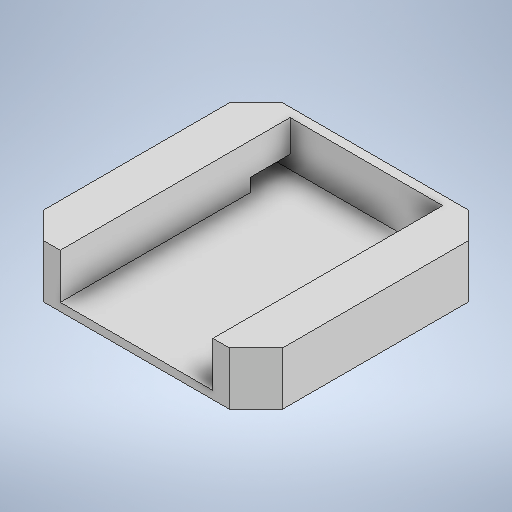
# Autodesk Inventor part: console case
Saved by Autodesk Inventor 2025.3 (Build 293356030, 356C)
## iProperties
Created: 2026-02-07
Part Number: console case
Material: Generic
Document SubType Name: Modeling
Designer: Adams
Density: 1 g/cm^3
Appearance: Default
Author: Adams
Autodesk Inventor part; units mm, degrees
ref_plane "YZ Plane" through (0, 0, 0) normal (1, 0, 0) x (0, 1, 0)
ref_plane "XZ Plane" through (0, 0, 0) normal (0, 1, 0) x (-1, 0, 0)
ref_plane "XY Plane" through (0, 0, 0) normal (0, 0, 1) x (1, 0, 0)
sketch "Sketch1" plane through (0, 0, 0) normal (0, 1, 0) x (-1, 0, 0)
  line L0 (28.75, 45) -> (-28.75, 45) construction
  line L1 (-28.75, 45) -> (-28.75, -41.6)
  line L2 (-28.75, -41.6) -> (28.75, -41.6)
  line L3 (28.75, -41.6) -> (28.75, 45)
  line L4 (28.75, 45) -> (-28.75, -41.6) construction
  line L5 (-28.75, 45) -> (28.75, -41.6) construction
  line L6 (45, 45) -> (-45, 45)
  line L7 (-45, 45) -> (-45, -45)
  line L8 (-45, -45) -> (45, -45)
  line L9 (45, -45) -> (45, 45)
  line L10 (45, 45) -> (-45, -45) construction
  line L11 (-45, 45) -> (45, -45) construction
  point P0 (0, 0)
  point P1 (0, 1.7)
  point P2 (28.75, 45)
  dimension "d0" = 57.5
  dimension "d1" = 86.6
  dimension "d2" = 90
  dimension "d3" = 90
  dimension "d4" = 0
  dimension "d5" = 0
  constraints: 24 end point, 4 midpoint, 4 parallel, 2 horizontal, 2 perpendicular
  measures "d0" distance of L2.end L1.end
  measures "d1" distance of L1.end L0.end
  measures "d2" distance of L8.end L7.end
  measures "d3" distance of L7.end L6.end
  measures "d4" distance between parallel lines of L6 L0
  measures "d5" horizontal distance of point (0, 1.7) point (0, 0)
extrude "Extrusion1" add sketch "Sketch1" against normal blind 3
extrude "Extrusion2" add sketch "Sketch1" along normal blind 17 contours L1 L2 L3 L6 L9 L8 L7
chamfer "Chamfer1" distance 10 angle 45 4 edges at (-45, 7, 45) (-45, 7, -45) (45, 7, -45) (45, 7, 45)
sketch "Sketch2" plane through (-45, -3, -35) normal (-1, 0, 0) x (0, 0, 1)
  line L0 (-6.6, 3) -> (-6.6, 20) projected
  line L1 (-6.6, 3) -> (8.4, 3)
  line L2 (8.4, 3) -> (8.4, 8)
  line L3 (8.4, 8) -> (-6.6, 8)
  line L4 (-6.6, 8) -> (-6.6, 3)
  point P0 (35, 3)
  dimension "d13" = 15
  dimension "d14" = 5
  constraints: 8 end point, 2 parallel, 1 horizontal, 1 perpendicular
  measures "d13" distance of L3.end L2.end
  measures "d14" distance of L2.end L1.end
extrude "Extrusion3" cut sketch "Sketch2" against normal blind 16.75
body "Solid1"
